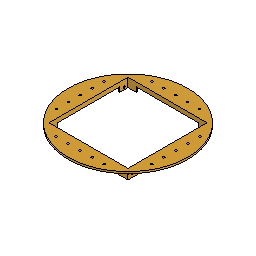
Plateau_3 (Autodesk Fusion 360 design; units mm, degrees)
Autodesk Fusion 360 part; units mm, degrees
sketch "Sketch1" plane through (0, 0, 0) normal (0, 0, 1) x (1, 0, 0)
  line L0 (82.6, -82.6) -> (67.4, -82.6)
  line L1 (-67.4, 67.4) -> (-82.6, 82.6) construction
  line L2 (82.6, 82.6) -> (82.6, 67.4)
  line L3 (67.4, -67.4) -> (82.6, -67.4)
  line L4 (82.6, 67.4) -> (67.4, 67.4)
  circle A0 centre (75, -75) radius 2.1
  line L5 (-67.4, -82.6) -> (-82.6, -82.6)
  circle A1 centre (0, 0) radius 125
  line L6 (67.4, 82.6) -> (82.6, 82.6)
  line L7 (-67.4, -67.4) -> (-67.4, -82.6)
  line L8 (-67.4, 82.6) -> (-67.4, 67.4)
  line L9 (82.6, -67.4) -> (82.6, -82.6)
  circle A2 centre (-75, 75) radius 2.1
  line L10 (-82.6, -82.6) -> (-82.6, -67.4)
  line L11 (-82.6, 67.4) -> (-82.6, 82.6)
  line L12 (-82.6, -67.4) -> (-67.4, -67.4)
  circle A3 centre (-75, -75) radius 2.1
  line L13 (-82.6, 82.6) -> (-67.4, 82.6)
  line L14 (-67.4, 67.4) -> (-82.6, 67.4)
  circle A4 centre (75, 75) radius 2.1
  line L15 (-82.6, 67.4) -> (-67.4, 82.6) construction
  line L16 (0, 0) -> (0, 36.3223) construction
  line L17 (67.4, 67.4) -> (67.4, 82.6)
  line L18 (0, 0) -> (-43.2001, 0) construction
  line L19 (67.4, -82.6) -> (67.4, -67.4)
  line L20 (-65.4, 84.6) -> (-65.4, 65.4)
  line L21 (-65.4, 65.4) -> (-84.6, 65.4)
  line L22 (-84.6, 65.4) -> (-84.6, 84.6)
  line L23 (-84.6, 84.6) -> (-65.4, 84.6)
  line L24 (84.6, 84.6) -> (84.6, 65.4)
  line L25 (65.4, 84.6) -> (84.6, 84.6)
  line L26 (84.6, 65.4) -> (65.4, 65.4)
  line L27 (65.4, 65.4) -> (65.4, 84.6)
  line L28 (-65.4, -65.4) -> (-65.4, -84.6)
  line L29 (-84.6, -65.4) -> (-65.4, -65.4)
  line L30 (-65.4, -84.6) -> (-84.6, -84.6)
  line L31 (-84.6, -84.6) -> (-84.6, -65.4)
  line L32 (84.6, -65.4) -> (84.6, -84.6)
  line L33 (65.4, -65.4) -> (84.6, -65.4)
  line L34 (84.6, -84.6) -> (65.4, -84.6)
  line L35 (65.4, -84.6) -> (65.4, -65.4)
  line L36 (-67.2001, 0) -> (-19.2001, 0) construction
  circle A5 centre (0, 0) radius 2.1
  circle A6 centre (-100, -100) radius 2.1
  circle A7 centre (-75, -100) radius 2.1
  circle A8 centre (-50, -100) radius 2.1
  circle A9 centre (-25, -100) radius 2.1
  circle A10 centre (0, -100) radius 2.1
  circle A11 centre (25, -100) radius 2.1
  circle A12 centre (50, -100) radius 2.1
  circle A13 centre (75, -100) radius 2.1
  circle A14 centre (100, -100) radius 2.1
  circle A15 centre (-100, -75) radius 2.1
  circle A16 centre (-75, -75) radius 2.1
  circle A17 centre (-50, -75) radius 2.1
  circle A18 centre (-25, -75) radius 2.1
  circle A19 centre (0, -75) radius 2.1
  circle A20 centre (25, -75) radius 2.1
  circle A21 centre (50, -75) radius 2.1
  circle A22 centre (75, -75) radius 2.1
  circle A23 centre (100, -75) radius 2.1
  circle A24 centre (-100, -50) radius 2.1
  circle A25 centre (-75, -50) radius 2.1
  circle A26 centre (-50, -50) radius 2.1
  circle A27 centre (-25, -50) radius 2.1
  circle A28 centre (0, -50) radius 2.1
  circle A29 centre (25, -50) radius 2.1
  circle A30 centre (50, -50) radius 2.1
  circle A31 centre (75, -50) radius 2.1
  circle A32 centre (100, -50) radius 2.1
  circle A33 centre (-100, -25) radius 2.1
  circle A34 centre (-75, -25) radius 2.1
  circle A35 centre (-50, -25) radius 2.1
  circle A36 centre (-25, -25) radius 2.1
  circle A37 centre (0, -25) radius 2.1
  circle A38 centre (25, -25) radius 2.1
  circle A39 centre (50, -25) radius 2.1
  circle A40 centre (75, -25) radius 2.1
  circle A41 centre (100, -25) radius 2.1
  circle A42 centre (-100, 0) radius 2.1
  circle A43 centre (-75, 0) radius 2.1
  circle A44 centre (-50, 0) radius 2.1
  circle A45 centre (-25, 0) radius 2.1
  circle A46 centre (25, 0) radius 2.1
  circle A47 centre (50, 0) radius 2.1
  circle A48 centre (75, 0) radius 2.1
  circle A49 centre (100, 0) radius 2.1
  circle A50 centre (-100, 25) radius 2.1
  circle A51 centre (-75, 25) radius 2.1
  circle A52 centre (-50, 25) radius 2.1
  circle A53 centre (-25, 25) radius 2.1
  circle A54 centre (0, 25) radius 2.1
  circle A55 centre (25, 25) radius 2.1
  circle A56 centre (50, 25) radius 2.1
  circle A57 centre (75, 25) radius 2.1
  circle A58 centre (100, 25) radius 2.1
  circle A59 centre (-100, 50) radius 2.1
  circle A60 centre (-75, 50) radius 2.1
  circle A61 centre (-50, 50) radius 2.1
  circle A62 centre (-25, 50) radius 2.1
  circle A63 centre (0, 50) radius 2.1
  circle A64 centre (25, 50) radius 2.1
  circle A65 centre (50, 50) radius 2.1
  circle A66 centre (75, 50) radius 2.1
  circle A67 centre (100, 50) radius 2.1
  circle A68 centre (-100, 75) radius 2.1
  circle A69 centre (-75, 75) radius 2.1
  circle A70 centre (-50, 75) radius 2.1
  circle A71 centre (-25, 75) radius 2.1
  circle A72 centre (0, 75) radius 2.1
  circle A73 centre (25, 75) radius 2.1
  circle A74 centre (50, 75) radius 2.1
  circle A75 centre (75, 75) radius 2.1
  circle A76 centre (100, 75) radius 2.1
  circle A77 centre (-100, 100) radius 2.1
  circle A78 centre (-75, 100) radius 2.1
  circle A79 centre (-50, 100) radius 2.1
  circle A80 centre (-25, 100) radius 2.1
  circle A81 centre (0, 100) radius 2.1
  circle A82 centre (25, 100) radius 2.1
  circle A83 centre (50, 100) radius 2.1
  circle A84 centre (75, 100) radius 2.1
  circle A85 centre (100, 100) radius 2.1
  line L37 (-75, -75) -> (-50, -75) construction
  line L38 (-67.4, 82.6) -> (67.4, 82.6)
  line L39 (82.6, 67.4) -> (82.6, -67.4)
  line L40 (67.4, -82.6) -> (-67.4, -82.6)
  line L41 (-82.6, -67.4) -> (-82.6, 67.4)
  point P0 (-75, 75)
  point P1 (-43.2001, 0)
  dimension "d3" = 150
  dimension "d4" = -150
  dimension "d7" = 150
  dimension "d8" = -150
  dimension "d9" = 15.2
  dimension "d10" = 15.2
  dimension "d11" = 75
  dimension "d12" = 75
  dimension "d13" = 250
  dimension "d16" = 4.2
  dimension "d15" = -2
  dimension "d73" = 4.2
  dimension "d76" = 25
  dimension "d77" = 25
  constraint horizontal L14
  constraint perpendicular L11 L14
  constraint parallel L13 L14
  constraint parallel L8 L11
  constraint coincident P0 L1
  constraint coincident P0 L15
  constraint coincident A1.centre L16.start
  constraint perpendicular L13 L16
  constraint perpendicular L16 L18
  constraint coincident P0 A2.centre
  constraint horizontal L36
  constraint midpoint P1 L36
  constraint coincident P1 L18.end
  constraint concentric A1 A5
  constraint coincident A3.centre A16.centre
  constraint coincident A17.centre L37.end
  measures "d9" distance of L1.end L8.start
  measures "d10" distance of L11.start L1.end
  measures "d11" vertical distance of A1.centre P0
  measures "d12" horizontal distance of A1.centre P0
  measures "d13" diameter of A1
  measures "d16" diameter of A2
  measures "d73" diameter of A5
extrude "Extrude1" add sketch "Sketch1" along normal blind 4 contours L0 L9 L32 L33 L34 L35 L39 L40 | L5 L10 L28 L29 L30 L31 L40 L41 | L2 L6 L24 L25 L26 L27 L38 L39 | L11 L13 L20 L21 L22 L23 L38 L41 | A1 A7 A13 A15 A23 A68 A76 A78 A84 | A1 A76 | A1 A23 | A1 A84 | A1 A13 | A1 A78 | A1 A7 | A1 A68 | A1 A15 picked at (99.4717, 74.5388) picked at (99.4717, -74.5388) picked at (74.5388, 99.4717) picked at (74.5388, -99.4717) picked at (-74.5525, 99.46) picked at (-74.5525, -99.46) picked at (-99.4166, 74.6108) picked at (-99.4166, -74.6108)
extrude "Extrude2" add sketch "Sketch1" against normal blind 15 contours L0 L9 L32 L33 L34 L35 L39 L40 | L5 L10 L28 L29 L30 L31 L40 L41 | L2 L6 L24 L25 L26 L27 L38 L39 | L11 L13 L20 L21 L22 L23 L38 L41
sketch "Sketch7" plane through (0, 0, 0) normal (0, 0, -1) x (1, 0, 0)
  circle A0 centre (0, 100) radius 2.1
  circle A1 centre (-100, 25) radius 2.1
  circle A2 centre (50, 100) radius 2.1
  circle A3 centre (100, 50) radius 2.1
  circle A4 centre (-100, 50) radius 2.1
  circle A5 centre (-25, -100) radius 2.1
  circle A6 centre (-100, -50) radius 2.1
  circle A7 centre (-50, -100) radius 2.1
  circle A8 centre (100, -50) radius 2.1
  circle A9 centre (50, -100) radius 2.1
  circle A10 centre (0, -100) radius 2.1
  circle A11 centre (25, -100) radius 2.1
  circle A12 centre (100, -25) radius 2.1
  circle A13 centre (100, 0) radius 2.1
  circle A14 centre (-100, -25) radius 2.1
  circle A15 centre (-50, 100) radius 2.1
  circle A16 centre (-25, 100) radius 2.1
  circle A17 centre (25, 100) radius 2.1
  circle A18 centre (-100, 0) radius 2.1
  circle A19 centre (100, 25) radius 2.1
  circle A20 centre (0, 0) radius 125
  line L0 (-82.6, -65.4) -> (-82.6, 65.4)
  line L1 (-65.4, 82.6) -> (65.4, 82.6)
  line L2 (82.6, 65.4) -> (82.6, -65.4)
  line L3 (65.4, -82.6) -> (-65.4, -82.6)
  line L4 (65.4, -84.6) -> (65.4, -82.6)
  line L5 (-65.4, -82.6) -> (-65.4, -84.6)
  line L6 (-65.4, -84.6) -> (-84.6, -84.6)
  line L7 (-84.6, -84.6) -> (-84.6, -65.4)
  line L8 (-84.6, -65.4) -> (-82.6, -65.4)
  line L9 (-82.6, 65.4) -> (-84.6, 65.4)
  line L10 (-84.6, 65.4) -> (-84.6, 84.6)
  line L11 (-84.6, 84.6) -> (-65.4, 84.6)
  line L12 (-65.4, 84.6) -> (-65.4, 82.6)
  line L13 (65.4, 82.6) -> (65.4, 84.6)
  line L14 (65.4, 84.6) -> (84.6, 84.6)
  line L15 (84.6, 84.6) -> (84.6, 65.4)
  line L16 (84.6, 65.4) -> (82.6, 65.4)
  line L17 (82.6, -65.4) -> (84.6, -65.4)
  line L18 (84.6, -65.4) -> (84.6, -84.6)
  line L19 (84.6, -84.6) -> (65.4, -84.6)
  line L20 (-65.4, -84.6) -> (65.4, -84.6)
  line L21 (65.4, -84.6) -> (65.4, -82.6)
  line L22 (65.4, -82.6) -> (-65.4, -82.6)
  line L23 (-65.4, -82.6) -> (-65.4, -84.6)
  line L24 (84.6, -65.4) -> (82.6, -65.4)
  line L25 (82.6, -65.4) -> (82.6, 65.4)
  line L26 (82.6, 65.4) -> (84.6, 65.4)
  line L27 (84.6, 65.4) -> (84.6, -65.4)
  line L28 (65.4, 82.6) -> (-65.4, 82.6)
  line L29 (-65.4, 82.6) -> (-65.4, 84.6)
  line L30 (-65.4, 84.6) -> (65.4, 84.6)
  line L31 (65.4, 84.6) -> (65.4, 82.6)
  line L32 (-82.6, 65.4) -> (-84.6, 65.4)
  line L33 (-84.6, 65.4) -> (-84.6, -65.4)
  line L34 (-84.6, -65.4) -> (-82.6, -65.4)
  line L35 (-82.6, -65.4) -> (-82.6, 65.4)
  constraint horizontal L20
  constraint vertical L21
  constraint horizontal L22
  constraint vertical L23
  constraint coincident L3.start L4.end
  constraint coincident L5.end L6.start
  constraint horizontal L24
  constraint vertical L25
  constraint horizontal L26
  constraint vertical L27
  constraint coincident L2.start L16.end
  constraint coincident L17.end L18.start
  constraint horizontal L28
  constraint vertical L29
  constraint horizontal L30
  constraint vertical L31
  constraint coincident L11.end L12.start
  constraint coincident L1.end L13.start
  constraint horizontal L32
  constraint vertical L33
  constraint horizontal L34
  constraint vertical L35
  constraint coincident L7.end L8.start
  constraint coincident L0.end L9.start
extrude "Extrude7" add sketch "Sketch7" along normal blind 5 contours L0 L8 L9 L32 L33 L34 L35 | L3 L4 L5 L20 L21 L22 L23 | L1 L12 L13 L28 L29 L30 L31 | L2 L16 L17 L24 L25 L26 L27
sketch "Sketch2" plane through (84.6, 0, 0) normal (1, 0, 0) x (0, 1, 0)
  line L0 (-65.4, -15) -> (-65.4, -5)
  line L1 (-84.6, -15) -> (-65.4, -15)
  line L2 (-84.6, 0) -> (-84.6, -15)
  line L3 (-84.6, 0) -> (-65.4, -15) construction
  line L4 (84.6, -15) -> (84.6, 0)
  line L5 (-84.6, -15) -> (-65.4, -15)
  line L6 (65.4, -5) -> (65.4, -15)
  line L7 (65.4, -5) -> (84.6, -15) construction
  circle A0 centre (-75, -7.5) radius 2.1
  circle A1 centre (75, -10) radius 2.1
  line L8 (-65.4, -5) -> (65.4, -5)
  line L9 (65.4, -5) -> (65.4, -15)
  line L10 (65.4, -15) -> (84.6, -15)
  line L11 (84.6, -15) -> (84.6, 0)
  line L12 (-84.6, 0) -> (-84.6, -15)
  line L13 (-65.4, -15) -> (-65.4, -5)
  line L14 (-65.4, -5) -> (65.4, -5)
  line L15 (65.4, -15) -> (84.6, -15)
  line L16 (84.6, 0) -> (-84.6, 0)
  line L17 (84.6, 0) -> (-84.6, 0)
  dimension "d24" = 4.2
  dimension "d25" = 4.2
  constraint coincident L2.start L3.start
  constraint coincident L0.start L1.end
  constraint coincident L6.start L7.start
  constraint coincident L4.start L7.end
  constraint midpoint L3 A0.centre
  constraint midpoint L7 A1.centre
  measures "d24" diameter of A0
  measures "d25" diameter of A1
extrude "Extrude3" cut sketch "Sketch2" against normal through all contours A0 | A1
fillet "Fillet6" radius 5 4 edges at (0, 84.6, 0) (84.6, 0, 0) (0, -84.6, 0) (-84.6, 0, 0)
sketch "Sketch3" plane through (0, 0, 4) normal (0, 0, 1) x (-1, 0, 0)
  circle A0 centre (0, 0) radius 125
  circle A1 centre (-90, 0) radius 70
  line L0 (0, 0) -> (-90, 0) construction
  circle A2 centre (-50, 75) radius 2.1
  circle A3 centre (-25, 75) radius 2.1
  circle A4 centre (0, 75) radius 2.1
  circle A5 centre (100, 50) radius 2.1
  circle A6 centre (75, 50) radius 2.1
  circle A7 centre (50, 50) radius 2.1
  circle A8 centre (25, 50) radius 2.1
  circle A9 centre (0, 50) radius 2.1
  circle A10 centre (-25, 50) radius 2.1
  circle A11 centre (-50, 50) radius 2.1
  circle A12 centre (-75, 50) radius 2.1
  circle A13 centre (-100, 50) radius 2.1
  circle A14 centre (100, 25) radius 2.1
  circle A15 centre (75, 25) radius 2.1
  circle A16 centre (0, 25) radius 2.1
  circle A17 centre (-50, 25) radius 2.1
  circle A18 centre (-75, 25) radius 2.1
  circle A19 centre (-100, 25) radius 2.1
  circle A20 centre (100, 0) radius 2.1
  circle A21 centre (75, 0) radius 2.1
  circle A22 centre (0, -25) radius 2.1
  circle A23 centre (75, -25) radius 2.1
  circle A24 centre (100, -25) radius 2.1
  circle A25 centre (-100, 0) radius 2.1
  circle A26 centre (-75, 0) radius 2.1
  circle A27 centre (-50, 0) radius 2.1
  circle A28 centre (-25, 0) radius 2.1
  circle A29 centre (-50, -25) radius 2.1
  circle A30 centre (-75, -25) radius 2.1
  circle A31 centre (-100, -25) radius 2.1
  circle A32 centre (100, -50) radius 2.1
  circle A33 centre (75, -50) radius 2.1
  circle A34 centre (50, -50) radius 2.1
  circle A35 centre (25, -50) radius 2.1
  circle A36 centre (0, -50) radius 2.1
  circle A37 centre (-25, -50) radius 2.1
  circle A38 centre (-50, -50) radius 2.1
  circle A39 centre (-75, -50) radius 2.1
  circle A40 centre (-100, -50) radius 2.1
  circle A41 centre (25, -75) radius 2.1
  circle A42 centre (0, -75) radius 2.1
  circle A43 centre (-25, -75) radius 2.1
  circle A44 centre (-50, -75) radius 2.1
  circle A45 centre (50, -100) radius 2.1
  circle A46 centre (25, -100) radius 2.1
  circle A47 centre (0, -100) radius 2.1
  circle A48 centre (-25, -100) radius 2.1
  circle A49 centre (-50, -100) radius 2.1
  circle A50 centre (50, 100) radius 2.1
  circle A51 centre (25, 100) radius 2.1
  circle A52 centre (0, 0) radius 2.1
  circle A53 centre (25, 75) radius 2.1
  circle A54 centre (-50, 100) radius 2.1
  circle A55 centre (0, 100) radius 2.1
  circle A56 centre (-25, 100) radius 2.1
  line L1 (-82.6, -67.4) -> (-67.4, -67.4)
  line L2 (-67.4, -67.4) -> (-67.4, -82.6)
  line L3 (-67.4, -82.6) -> (-82.6, -82.6)
  line L4 (-82.6, -82.6) -> (-82.6, -67.4)
  line L5 (67.4, -82.6) -> (67.4, -67.4)
  line L6 (67.4, -67.4) -> (82.6, -67.4)
  line L7 (82.6, -67.4) -> (82.6, -82.6)
  line L8 (82.6, -82.6) -> (67.4, -82.6)
  line L9 (-82.6, 82.6) -> (-67.4, 82.6)
  line L10 (-67.4, 82.6) -> (-67.4, 67.4)
  line L11 (-67.4, 67.4) -> (-82.6, 67.4)
  line L12 (-82.6, 67.4) -> (-82.6, 82.6)
  line L13 (82.6, 82.6) -> (82.6, 67.4)
  line L14 (82.6, 67.4) -> (67.4, 67.4)
  line L15 (67.4, 67.4) -> (67.4, 82.6)
  line L16 (67.4, 82.6) -> (82.6, 82.6)
  line L17 (-39, 47.9479) -> (-39, -47.9479)
  circle A57 centre (-25, -25) radius 2.1
  circle A58 centre (-25, 25) radius 2.1
  line L18 (65.4, -69) -> (65.4, -81)
  line L19 (65.4, -81) -> (53.4, -81)
  arc A59 (53.4, -69) -> (53.4, -81) centre (53.4, -75) ccw
  line L20 (53.4, -69) -> (65.4, -69)
  line L21 (65.4, 81) -> (65.4, 69)
  line L22 (65.4, 69) -> (53.4, 69)
  arc A60 (53.4, 81) -> (53.4, 69) centre (53.4, 75) ccw
  line L23 (53.4, 81) -> (65.4, 81)
  circle A61 centre (25, -25) radius 2.1
  circle A62 centre (50, 25) radius 2.1
  circle A63 centre (25, 0) radius 2.1
  circle A64 centre (50, -25) radius 2.1
  circle A65 centre (50, 0) radius 2.1
  circle A66 centre (25, 25) radius 2.1
  dimension "d29" = 140
  dimension "d31" = 90
  dimension "d79" = 14
  constraint coincident A0.centre L0.start
  constraint coincident A1.centre L0.end
  constraint horizontal L0
  constraint coincident A1 L17.start
  constraint coincident A1 L17.end
  constraint perpendicular L0 L17
  measures "d29" diameter of A1
  measures "d31" distance of A0.centre A1.centre
  measures "d79" distance of A28.centre L17
extrude "Extrude5" [suppressed]
fillet "Fillet4" [suppressed]
copy_body "Body->Comp1" [suppressed] in component "Mignon_Plateau_oeil"
sketch "Sketch8" plane through (0, 0, 0) normal (0, 0, -1) x (1, 0, 0)
  arc A0 (49.5556, -57.1336) -> (56.3839, -61.4) centre (90, 0) ccw
  arc A1 (39, -36.7287) -> (49.5556, -57.1336) centre (64, -36.7287) ccw
  line L0 (39, -36.7287) -> (39, 36.7287)
  arc A2 (49.5556, 57.1336) -> (39, 36.7287) centre (64, 36.7287) ccw
  arc A3 (56.3839, 61.4) -> (49.5556, 57.1336) centre (90, 0) ccw
  line L1 (56.3839, 61.4) -> (-9.5, 61.4)
  line L2 (-9.5, 61.4) -> (-9.5, -61.4)
  line L3 (-9.5, -61.4) -> (56.3839, -61.4)
  circle A4 centre (25, 50) radius 2.1
  circle A5 centre (0, 25) radius 2.1
  circle A6 centre (25, 25) radius 2.1
  circle A7 centre (25, -25) radius 2.1
  circle A8 centre (25, -50) radius 2.1
  circle A9 centre (0, -50) radius 2.1
  circle A10 centre (0, -25) radius 2.1
  circle A11 centre (25, 0) radius 2.1
  circle A12 centre (0, 50) radius 2.1
  circle A13 centre (0, 0) radius 2.1
  line L4 (-12, -61.4) -> (-12, 61.4)
  line L5 (-12, -7) -> (0, -7)
  line L6 (0, -7) -> (0, 7)
  line L7 (0, 7) -> (-12, 7)
  line L8 (-12, 7) -> (-12, -7)
  dimension "d187" = 14
  constraint horizontal L5
  constraint vertical L6
  constraint horizontal L7
  constraint vertical L8
  constraint coincident L4 L5.start
  constraint coincident A13.centre L6
  constraint midpoint A13.centre L6
  measures "d187" distance of L5.end L6.end
extrude "Extrude2'" [suppressed] in component "Mignon_Plateau_oeil"
move_body "Move1" [suppressed] in component "Mignon_Plateau_oeil"
ref_plane "WorkPlane1" through (64.7917, 50.1917, 13.5) normal (0, -1, 0) x (-1, 0, 0)
ref_plane "WorkPlane2" through (50.1917, 41.3417, 17.5) normal (-1, 0, 0) x (0, -1, 0)
split "Split1" [suppressed] in component "Mignon_Plateau_oeil"
split "Split2" [suppressed] in component "Mignon_Plateau_oeil"
named bodies: "Plateau_3", "Mignon_Plateau_oeil", "Mignon_Plateau_oeil (1)", "Mignon_Plateau_oeil (2)"
